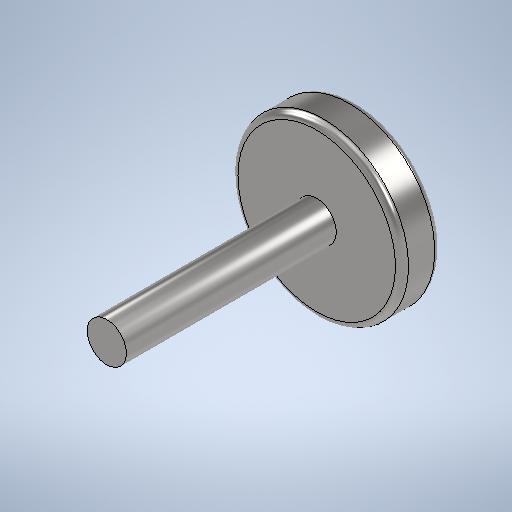
# Autodesk Inventor part: handle
Saved by Autodesk Inventor 2025 (Build 290162010, 162A)
## iProperties
Created: 2024-06-06
Part Number: handle
Material: Stahl, weich
Document SubType Name: Modeling
Designer: ffogue
Density: 7.85 g/cm^3
Appearance: Halbpoliert
Author: ffogue
Autodesk Inventor part; units mm, degrees
ref_plane "YZ Plane" through (0, 0, 0) normal (1, 0, 0) x (0, 1, 0)
ref_plane "XZ Plane" through (0, 0, 0) normal (0, 1, 0) x (-1, 0, 0)
ref_plane "XY Plane" through (0, 0, 0) normal (0, 0, 1) x (1, 0, 0)
sketch "Skizze1" plane through (0, 0, 0) normal (0, 1, 0) x (-1, 0, 0)
  circle A0 centre (0, 0) radius 13
  dimension "d0" = 26
  constraints: 1 centre point, 1 coincident
  measures "d0" diameter of A0
extrude "Extrusion1" add sketch "Skizze1" along normal blind 6
sketch "Skizze2" plane through (0, 0, 0) normal (0, -1, 0) x (1, 0, 0)
  circle A0 centre (0, 0) radius 3
  dimension "d3" = 6
  constraints: 1 centre point, 1 coincident
  measures "d3" diameter of A0
extrude "Extrusion2" add sketch "Skizze2" along normal blind 32
sketch "Skizze3" plane through (0, 0, 0) normal (0, 1, 0) x (1, 0, 0)
  circle A0 centre (-9.5, 0) radius 1.5
  point P0 (0, 0)
  dimension "d6" = 3
  dimension "d7" = 9.5
  constraints: 1 centre point, 1 horizontal alignment
  measures "d6" diameter of A0
  measures "d7" distance of point (0, 0) A0.centre
extrude "Extrusion3" add sketch "Skizze3" along normal blind 13.5
fillet "Rundung1" radius 1 2 edges at (13, 0, 0) (13, 6, 0)
